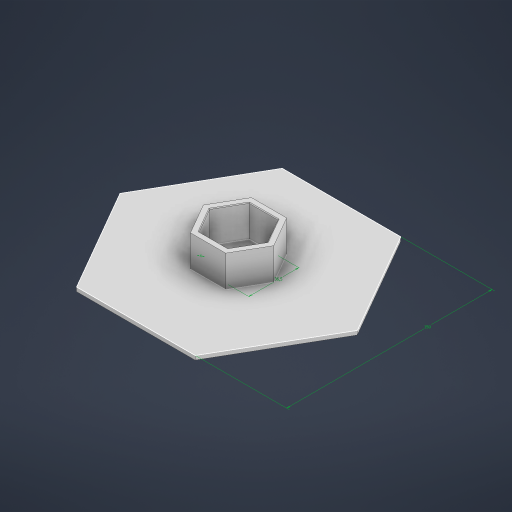
# Autodesk Inventor part: staender_tisch
Saved by Autodesk Inventor 2023 (Build 270158000, 158)
## iProperties
Created: 2022-08-10
Part Number: staender_tisch
Material: Generic
Document SubType Name: Modeling
Designer: bananenbrot
Density: 1 g/cm^3
Appearance: Default
Author: bananenbrot
Autodesk Inventor part; units mm, degrees
ref_plane "YZ Plane" through (0, 0, 0) normal (1, 0, 0) x (0, 1, 0)
ref_plane "XZ Plane" through (0, 0, 0) normal (0, 1, 0) x (-1, 0, 0)
ref_plane "XY Plane" through (0, 0, 0) normal (0, 0, 1) x (1, 0, 0)
sketch "Sketch1" plane through (0, 0, 0) normal (0, 1, 0) x (-1, 0, 0)
  line L0 (21.0733, 0) -> (10.5366, -18.25)
  line L1 (10.5366, -18.25) -> (-10.5366, -18.25)
  line L2 (-10.5366, -18.25) -> (-21.0733, 0)
  line L3 (-21.0733, 0) -> (-10.5366, 18.25)
  line L4 (-10.5366, 18.25) -> (10.5366, 18.25)
  line L5 (10.5366, 18.25) -> (21.0733, 0)
  line L6 (25.6921, 0) -> (12.846, -22.25)
  line L7 (12.846, -22.25) -> (-12.846, -22.25)
  line L8 (-12.846, -22.25) -> (-25.6921, 0)
  line L9 (-25.6921, 0) -> (-12.846, 22.25)
  line L10 (-12.846, 22.25) -> (12.846, 22.25)
  line L11 (12.846, 22.25) -> (25.6921, 0)
  line L12 (86.6025, 0) -> (43.3013, -75)
  line L13 (43.3013, -75) -> (-43.3013, -75)
  line L14 (-43.3013, -75) -> (-86.6025, 0)
  line L15 (-86.6025, 0) -> (-43.3013, 75)
  line L16 (-43.3013, 75) -> (43.3013, 75)
  line L17 (43.3013, 75) -> (86.6025, 0)
  point P0 (0, 0)
  point P1 (0, 0)
  dimension "d0" = 36.5
  dimension "d1" = 4
  dimension "d2" = 150
  constraints: 36 end point, 1 coincident, 1 horizontal alignment, 23 other
  measures "d0" distance between parallel lines of L1 L4
  measures "d1" distance between parallel lines of L5 L11
  measures "d2" distance between parallel lines of L13 L16
extrude "Extrusion1" add sketch "Sketch1" along normal blind 23 contours L6 L7 L8 L9 L10 L11
extrude "Extrusion2" add sketch "Sketch1" against normal blind 3 contours L0 L1 L2 L3 L4 L5 | L6 L7 L8 L9 L10 L11 | L12 L13 L14 L15 L16 L17
sketch "Sketch2" plane through (0, 0, 0) normal (0, 1, 0) x (1, 0, 0)
  circle A0 centre (0, 0) radius 9.85
  circle A1 centre (0, 0) radius 9
  dimension "d7" = 19.7
  dimension "d8" = 18
  constraints: 2 centre point, 2 coincident
  measures "d7" diameter of A0
  measures "d8" diameter of A1
extrude "Extrusion3" [suppressed]
chamfer "Chamfer1" distance 0.5 angle 45 6 edges at (0, 23, 18.25) (-15.805, 23, 9.125) (-15.805, 23, -9.125) (0, 23, -18.25) (15.805, 23, -9.125) (15.805, 23, 9.125)
chamfer "Chamfer2" [suppressed]
body "Solid1"
